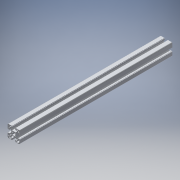
# Autodesk Inventor part: Table Leg
Saved by Autodesk Inventor 2019.4 (Build 234330000, 330)
## iProperties
Created: 2005-02-27
Part Number: Table Leg
Project: 40
User Status: FOR INFORMATION
Material: SolidWorks Materials|6061 Alloy
Description: 40X40L
Document SubType Name: Modeling
Designer: admin
Density: 2.7 g/cm^3
Appearance: 229,234,237
Sending System: SolidWorks 2016
Last Author: Steve
Last Saved: 2016-08-04
Part Number: 3 842 993 120
Vendor Name: BOSCH REXROTH
Left Finish: NONE
Length: 200
UNIT_OF_MEASURE: - none -
Right Finish: NONE
Author: pdmwadmin
Revision Number: A
Autodesk Inventor part; units mm, degrees
ref_plane "YZ Plane" through (0, 0, 0) normal (1, 0, 0) x (0, 1, 0)
ref_plane "XZ Plane" through (0, 0, 0) normal (0, 1, 0) x (-1, 0, 0)
ref_plane "XY Plane" through (0, 0, 0) normal (0, 0, 1) x (1, 0, 0)
sketch "Sketch1" plane through (6.0858, -7.5, 0) normal (0, 0, -1) x (-1, 0, 0)
  line L0 (0.2858, -11) -> (0.2858, -12.5) projected
  line L1 (1.0858, -11) -> (0.2858, -11) projected
  line L2 (1.0858, -6.5) -> (1.0858, -11) projected
  line L3 (-3.9642, -6.5) -> (1.0858, -6.5) projected
  line L4 (-3.9642, -3.9642) -> (-3.9642, -6.5) projected
  line L5 (0, 0) -> (-3.9642, -3.9642) projected
  line L6 (12.1716, 0) -> (0, 0) projected
  line L7 (16.1358, -3.9642) -> (12.1716, 0) projected
  line L8 (16.1358, -6.5) -> (16.1358, -3.9642) projected
  line L9 (11.0858, -6.5) -> (16.1358, -6.5) projected
  line L10 (11.0858, -11) -> (11.0858, -6.5) projected
  line L11 (11.8858, -11) -> (11.0858, -11) projected
  line L12 (11.8858, -12.5) -> (11.8858, -11) projected
  line L13 (23.0858, -12.5) -> (11.8858, -12.5) projected
  arc A0 (23.0858, -12.5) -> (26.0858, -9.5) centre (23.0858, -9.5) ccw projected
  line L14 (26.0858, 1.7) -> (26.0858, -9.5) projected
  line L15 (24.5858, 1.7) -> (26.0858, 1.7) projected
  line L16 (24.5858, 2.5) -> (24.5858, 1.7) projected
  line L17 (20.0858, 2.5) -> (24.5858, 2.5) projected
  line L18 (20.0858, -2.55) -> (20.0858, 2.5) projected
  line L19 (17.55, -2.55) -> (20.0858, -2.55) projected
  line L20 (13.5858, 1.4142) -> (17.55, -2.55) projected
  line L21 (13.5858, 13.5858) -> (13.5858, 1.4142) projected
  line L22 (17.55, 17.55) -> (13.5858, 13.5858) projected
  line L23 (20.0858, 17.55) -> (17.55, 17.55) projected
  line L24 (20.0858, 12.5) -> (20.0858, 17.55) projected
  line L25 (24.5858, 12.5) -> (20.0858, 12.5) projected
  line L26 (24.5858, 13.3) -> (24.5858, 12.5) projected
  line L27 (26.0858, 13.3) -> (24.5858, 13.3) projected
  line L28 (26.0858, 24.5) -> (26.0858, 13.3) projected
  arc A1 (26.0858, 24.5) -> (23.0858, 27.5) centre (23.0858, 24.5) ccw projected
  line L29 (11.8858, 27.5) -> (23.0858, 27.5) projected
  line L30 (11.8858, 26) -> (11.8858, 27.5) projected
  line L31 (11.0858, 26) -> (11.8858, 26) projected
  line L32 (11.0858, 21.5) -> (11.0858, 26) projected
  line L33 (16.1358, 21.5) -> (11.0858, 21.5) projected
  line L34 (16.1358, 18.9642) -> (16.1358, 21.5) projected
  line L35 (12.1716, 15) -> (16.1358, 18.9642) projected
  line L36 (0, 15) -> (12.1716, 15) projected
  line L37 (-3.9642, 18.9642) -> (0, 15) projected
  line L38 (-3.9642, 21.5) -> (-3.9642, 18.9642) projected
  line L39 (1.0858, 21.5) -> (-3.9642, 21.5) projected
  line L40 (1.0858, 26) -> (1.0858, 21.5) projected
  line L41 (0.2858, 26) -> (1.0858, 26) projected
  line L42 (0.2858, 27.5) -> (0.2858, 26) projected
  line L43 (-10.9142, 27.5) -> (0.2858, 27.5) projected
  arc A2 (-10.9142, 27.5) -> (-13.9142, 24.5) centre (-10.9142, 24.5) ccw projected
  line L44 (-13.9142, 13.3) -> (-13.9142, 24.5) projected
  line L45 (-12.4142, 13.3) -> (-13.9142, 13.3) projected
  line L46 (-12.4142, 12.5) -> (-12.4142, 13.3) projected
  line L47 (-7.9142, 12.5) -> (-12.4142, 12.5) projected
  line L48 (-7.9142, 17.55) -> (-7.9142, 12.5) projected
  line L49 (-5.3784, 17.55) -> (-7.9142, 17.55) projected
  line L50 (-1.4142, 13.5858) -> (-5.3784, 17.55) projected
  line L51 (-1.4142, 1.4142) -> (-1.4142, 13.5858) projected
  line L52 (-5.3784, -2.55) -> (-1.4142, 1.4142) projected
  line L53 (-7.9142, -2.55) -> (-5.3784, -2.55) projected
  line L54 (-7.9142, 2.5) -> (-7.9142, -2.55) projected
  line L55 (-12.4142, 2.5) -> (-7.9142, 2.5) projected
  line L56 (-12.4142, 1.7) -> (-12.4142, 2.5) projected
  line L57 (-13.9142, 1.7) -> (-12.4142, 1.7) projected
  line L58 (-13.9142, -9.5) -> (-13.9142, 1.7) projected
  arc A3 (-13.9142, -9.5) -> (-10.9142, -12.5) centre (-10.9142, -9.5) ccw projected
  line L59 (0.2858, -12.5) -> (-10.9142, -12.5) projected
  arc A4 (-12.4142, 17) -> (-9.4142, 17) centre (-10.9142, 17) ccw projected
  line L60 (-12.4142, 17) -> (-12.4142, 22) projected
  line L61 (-12.4142, 22) -> (-11.1642, 22) projected
  arc A5 (-8.4142, 24.75) -> (-11.1642, 22) centre (-8.4142, 22) ccw projected
  line L62 (-8.4142, 24.75) -> (-8.4142, 26) projected
  line L63 (-8.4142, 26) -> (-3.4142, 26) projected
  arc A6 (-3.4142, 23) -> (-3.4142, 26) centre (-3.4142, 24.5) ccw projected
  line L64 (-3.4142, 23) -> (-5.6642, 23) projected
  line L65 (-5.6642, 23) -> (-5.6642, 22) projected
  arc A7 (-8.4142, 19.25) -> (-5.6642, 22) centre (-8.4142, 22) ccw projected
  line L66 (-8.4142, 19.25) -> (-9.4142, 19.25) projected
  line L67 (-9.4142, 19.25) -> (-9.4142, 17) projected
  arc A8 (8.084, 12.0833) -> (4.0875, 12.0833) centre (6.0858, 7.5) ccw projected
  line L68 (8.084, 12.0833) -> (8.4837, 13) projected
  line L69 (8.4837, 13) -> (11.5858, 13) projected
  line L70 (11.5858, 13) -> (11.5858, 9.8979) projected
  line L71 (11.5858, 9.8979) -> (10.6691, 9.4983) projected
  arc A9 (10.6691, 5.5017) -> (10.6691, 9.4983) centre (6.0858, 7.5) ccw projected
  line L72 (10.6691, 5.5017) -> (11.5858, 5.1021) projected
  line L73 (11.5858, 5.1021) -> (11.5858, 2) projected
  line L74 (11.5858, 2) -> (8.4837, 2) projected
  line L75 (8.4837, 2) -> (8.084, 2.9167) projected
  arc A10 (4.0875, 2.9167) -> (8.084, 2.9167) centre (6.0858, 7.5) ccw projected
  line L76 (4.0875, 2.9167) -> (3.6879, 2) projected
  line L77 (3.6879, 2) -> (0.5858, 2) projected
  line L78 (0.5858, 2) -> (0.5858, 5.1021) projected
  line L79 (0.5858, 5.1021) -> (1.5025, 5.5017) projected
  arc A11 (1.5025, 9.4983) -> (1.5025, 5.5017) centre (6.0858, 7.5) ccw projected
  line L80 (1.5025, 9.4983) -> (0.5858, 9.8979) projected
  line L81 (0.5858, 9.8979) -> (0.5858, 13) projected
  line L82 (0.5858, 13) -> (3.6879, 13) projected
  line L83 (3.6879, 13) -> (4.0875, 12.0833) projected
  arc A12 (17.8358, 22) -> (20.5858, 19.25) centre (20.5858, 22) ccw projected
  line L84 (17.8358, 22) -> (17.8358, 23) projected
  line L85 (17.8358, 23) -> (15.5858, 23) projected
  arc A13 (15.5858, 26) -> (15.5858, 23) centre (15.5858, 24.5) ccw projected
  line L86 (15.5858, 26) -> (20.5858, 26) projected
  line L87 (20.5858, 26) -> (20.5858, 24.75) projected
  arc A14 (23.3358, 22) -> (20.5858, 24.75) centre (20.5858, 22) ccw projected
  line L88 (23.3358, 22) -> (24.5858, 22) projected
  line L89 (24.5858, 22) -> (24.5858, 17) projected
  arc A15 (21.5858, 17) -> (24.5858, 17) centre (23.0858, 17) ccw projected
  line L90 (21.5858, 17) -> (21.5858, 19.25) projected
  line L91 (21.5858, 19.25) -> (20.5858, 19.25) projected
  arc A16 (24.5858, -2) -> (21.5858, -2) centre (23.0858, -2) ccw projected
  line L92 (24.5858, -2) -> (24.5858, -7) projected
  line L93 (24.5858, -7) -> (23.3358, -7) projected
  arc A17 (20.5858, -9.75) -> (23.3358, -7) centre (20.5858, -7) ccw projected
  line L94 (20.5858, -9.75) -> (20.5858, -11) projected
  line L95 (20.5858, -11) -> (15.5858, -11) projected
  arc A18 (15.5858, -8) -> (15.5858, -11) centre (15.5858, -9.5) ccw projected
  line L96 (15.5858, -8) -> (17.8358, -8) projected
  line L97 (17.8358, -8) -> (17.8358, -7) projected
  arc A19 (20.5858, -4.25) -> (17.8358, -7) centre (20.5858, -7) ccw projected
  line L98 (20.5858, -4.25) -> (21.5858, -4.25) projected
  line L99 (21.5858, -4.25) -> (21.5858, -2) projected
  arc A20 (-5.6642, -7) -> (-8.4142, -4.25) centre (-8.4142, -7) ccw projected
  line L100 (-5.6642, -7) -> (-5.6642, -8) projected
  line L101 (-5.6642, -8) -> (-3.4142, -8) projected
  arc A21 (-3.4142, -11) -> (-3.4142, -8) centre (-3.4142, -9.5) ccw projected
  line L102 (-3.4142, -11) -> (-8.4142, -11) projected
  line L103 (-8.4142, -11) -> (-8.4142, -9.75) projected
  arc A22 (-11.1642, -7) -> (-8.4142, -9.75) centre (-8.4142, -7) ccw projected
  line L104 (-11.1642, -7) -> (-12.4142, -7) projected
  line L105 (-12.4142, -7) -> (-12.4142, -2) projected
  arc A23 (-9.4142, -2) -> (-12.4142, -2) centre (-10.9142, -2) ccw projected
  line L106 (-9.4142, -2) -> (-9.4142, -4.25) projected
  line L107 (-9.4142, -4.25) -> (-8.4142, -4.25) projected
extrude "Extrusion1" add sketch "Sketch1" against normal blind 500
body "Solid1"
